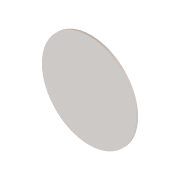
# Autodesk Inventor part: Filter
Saved by Autodesk Inventor 2021 (Build 250183000, 183)
## iProperties
Created: 2023-02-07
Part Number: Filter
Material: Glass
Document SubType Name: Modeling
Designer: nvladi
Density: 2.18 g/cm^3
Appearance: Clear
Author: nvladi
Autodesk Inventor part; units mm, degrees
ref_plane "YZ Plane" through (0, 0, 0) normal (1, 0, 0) x (0, 1, 0)
ref_plane "XZ Plane" through (0, 0, 0) normal (0, 1, 0) x (-1, 0, 0)
ref_plane "XY Plane" through (0, 0, 0) normal (0, 0, 1) x (1, 0, 0)
sketch "Sketch1" plane through (0, 0, 0) normal (0, 0, 1) x (1, 0, 0)
  circle A0 centre (0, 0) radius 25
  dimension "d0" = 50
  constraints: 1 centre point, 1 coincident
  measures "d0" diameter of A0
extrude "Extrusion1" add sketch "Sketch1" along normal blind 1
body "Solid1"
